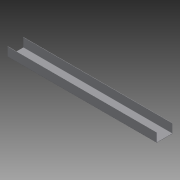
# Autodesk Inventor part: Część5
Saved by Autodesk Inventor 2014 (Build 180170000, 170)
## iProperties
Created: 2013-12-25
Part Number: Część5
Material: Ogólny
Document SubType Name: Sheet Metal
Designer: Kuba
Density: 1 g/cm^3
Sheet Metal Rule: Default_mm
Appearance: Domyślna
Author: Kuba
Autodesk Inventor part; units mm, degrees
note: some values were not read from the file. Chosen so that the rebuilt part matches the saved one: flange form of "Płyta1".
ref_plane "YZ Plane" through (0, 0, 0) normal (1, 0, 0) x (0, 1, 0)
ref_plane "XZ Plane" through (0, 0, 0) normal (0, 1, 0) x (-1, 0, 0)
ref_plane "XY Plane" through (0, 0, 0) normal (0, 0, 1) x (1, 0, 0)
sketch "Szkic1" plane through (0, 0, 0) normal (1, 0, 0) x (0, 1, 0)
  line L0 (-19.507, 0) -> (22.493, 0)
  line L1 (0, -18.291) -> (0, 5.509)
  line L2 (16.493, -14.891) -> (-13.507, -14.891)
  line L3 (-13.507, -14.891) -> (-13.507, 2.109)
  line L4 (16.493, -14.891) -> (16.493, 2.109)
  point P0 (0, 0)
  dimension "d1" = 30
  dimension "d2" = 17
  dimension "d3" = 17
  measures "d1" distance of L2.start L2.end
  measures "d2" distance of L2.end L3.end
  measures "d3" distance of L2.start L4.end
contour flange "Kołnierz z profilu1" sketch "Szkic1" thickness 0.5 bend radius 0.5 width 184 along (1, 0, 0) mid plane no both sides no wall seen from (0, 16.493, -6.391) lies toward (0, -1, 0) curves L4 L2 L3
bend "Gięcie1"
corner "Narożnik1"
equation "\"d3\" = d2"
equation "\"d4\" = SzerokośćGięciaPodcięcia"
equation "\"d5\" = GłębokośćGięciaPodcięcia"
equation "\"d6\" = MinimalnaPozostałość"
equation "\"d7\" = PromieńGięcia"
equation "\"d9\" = PromieńGięcia"
equation "\"d11\" = RozmiarPodcięciaNarożnika"
equation "\"d12\" = Wielk_odstępu"
equation "\"d13\" = Rozmiar_promienia_Jacobiego"
equation "\"PromieńGięcia\" = Grubość"
equation "\"SzerokośćGięciaPodcięcia\" = Grubość"
equation "\"GłębokośćGięciaPodcięcia\" = 0.5 * Grubość"
equation "\"RozmiarPodcięciaNarożnika\" = 4 * Grubość"
equation "\"MinimalnaPozostałość\" = 2 * Grubość"
equation "\"PromieńPrzejścia\" = PromieńGięcia"
equation "\"Rozmiar_promienia_Jacobiego\" = PromieńGięcia"
equation "\"Wielk_odstępu\" = Grubość"
equation "\"Grubość\" = 0.5"
